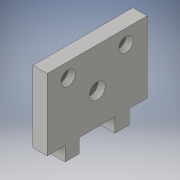
# Autodesk Inventor part: Far End Cap
Saved by Autodesk Inventor 2016 (Build 200138000, 138)
## iProperties
Created: 2016-04-25
Part Number: Far End Cap
Material: Generic
Document SubType Name: Modeling
Designer: rubenjm
Density: 1 g/cm^3
Appearance: Default
Author: rubenjm
Autodesk Inventor part; units mm, degrees
ref_plane "YZ Plane" through (0, 0, 0) normal (1, 0, 0) x (0, 1, 0)
ref_plane "XZ Plane" through (0, 0, 0) normal (0, 1, 0) x (-1, 0, 0)
ref_plane "XY Plane" through (0, 0, 0) normal (0, 0, 1) x (1, 0, 0)
sketch "Sketch1" plane through (0, 0, 0) normal (1, 0, 0) x (0, 1, 0)
  circle A0 centre (27.94, -44.6106) radius 6.985 construction
  circle A1 centre (50.8, -18.5683) radius 6.35 construction
  line L0 (63.5, 0) -> (50.8, 0) construction
  line L1 (50.8, 0) -> (50.8, -12.7) construction
  line L2 (50.8, -12.7) -> (63.5, -12.7) construction
  line L3 (63.5, -12.7) -> (63.5, 0) construction
  circle A2 centre (50.8, -70.0106) radius 6.35 construction
  line L4 (27.94, -31.779) -> (39.0525, -38.1948) construction
  line L5 (39.0525, -38.1948) -> (39.0525, -51.0264) construction
  line L6 (39.0525, -51.0264) -> (27.94, -57.4422) construction
  line L7 (27.94, -57.4422) -> (16.8275, -51.0264) construction
  line L8 (16.8275, -51.0264) -> (16.8275, -38.1948) construction
  line L9 (63.5, 0) -> (0, 0)
  line L10 (0, -88.9) -> (63.5, -88.9)
  line L11 (63.5, -88.9) -> (63.5, 0)
  line L12 (0, -44.45) -> (27.94, -44.45) construction
  line L13 (0, -44.45) -> (27.94, -44.45) construction
  line L14 (27.94, -31.779) -> (16.8275, -38.1948) construction
  line L15 (0, -44.45) -> (63.5, -44.45) construction
  line L16 (0, -44.45) -> (0, -60.325) construction
  line L17 (0, -44.45) -> (15.875, -44.45) construction
  line L18 (0, -60.325) -> (-12.7, -60.325)
  line L19 (-12.7, -60.325) -> (-12.7, -73.025)
  line L20 (-12.7, -73.025) -> (0, -73.025)
  line L21 (0, -44.45) -> (0, -28.575) construction
  line L22 (0, -28.575) -> (-12.7, -28.575)
  line L23 (-12.7, -28.575) -> (-12.7, -15.875)
  line L24 (-12.7, -15.875) -> (0, -15.875)
  line L25 (0, 0) -> (0, -15.875)
  line L26 (0, -28.575) -> (0, -60.325)
  line L27 (0, -73.025) -> (0, -88.9)
  point P0 (0, 0)
  point P1 (0, -12.8606)
  dimension "d13" = 88.9
  dimension "d14" = 63.5
  dimension "d15" = 15.875
  dimension "d16" = 90
  dimension "d17" = 12.7
  dimension "d18" = 12.7
  constraints: 56 end point, 7 parallel, 6 horizontal, 5 perpendicular, 4 symmetric about line, 3 centre point, 3 midpoint, 2 equal length, 1 point on line, 1 vertical
  measures "d13" distance of L10.end L0.start
  measures "d14" distance of L10.start L10.end
  measures "d15" distance of L15.start L16.end
  measures "d16" angle of L16 L17
  measures "d17" distance of L20.end L19.end
  measures "d18" distance of L19.end L18.end
extrude "Extrusion2" add sketch "Sketch1" along normal blind 12.7
sketch "Sketch2" plane through (12.7, 0, 0) normal (1, 0, 0) x (0, 0, -1)
  circle A0 centre (44.6106, 27.94) radius 6.985
  circle A1 centre (18.5683, 50.8) radius 6.35
  line L0 (0, 50.8) -> (12.7, 50.8) construction
  line L1 (12.7, 50.8) -> (12.7, 63.5) construction
  circle A2 centre (70.0106, 50.8) radius 6.35
  line L2 (31.779, 27.94) -> (38.1948, 39.0525) construction
  line L3 (38.1948, 39.0525) -> (51.0264, 39.0525) construction
  line L4 (51.0264, 39.0525) -> (57.4422, 27.94) construction
  line L5 (57.4422, 27.94) -> (51.0264, 16.8275) construction
  line L6 (51.0264, 16.8275) -> (38.1948, 16.8275) construction
  line L7 (44.45, 0) -> (44.45, 27.94) construction
  line L8 (44.45, 0) -> (44.45, 27.94) construction
  line L9 (31.779, 27.94) -> (38.1948, 16.8275) construction
  line L10 (44.45, 0) -> (44.45, 15.875) construction
  line L11 (88.9, 0) -> (88.9, 63.5) construction
  line L12 (0, 0) -> (88.9, 0) construction
  line L13 (28.575, 0) -> (60.325, 0) construction
  line L14 (44.45, 0) -> (44.45, 63.5) construction
  line L15 (88.9, 63.5) -> (0, 63.5) construction
  constraints: 26 end point, 3 centre point, 2 midpoint, 1 collinear, 1 horizontal, 1 point on line
extrude "Extrusion3" cut sketch "Sketch2" against normal blind 6.35
body "Solid2"
